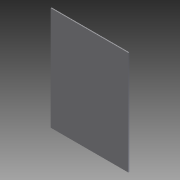
# Autodesk Inventor part: PCB
Saved by Autodesk Inventor 2012 (Build 160160000, 160)
## iProperties
Created: 2017-04-26
Part Number: PCB
Material: Default
Document SubType Name: Modeling
Designer: Brandon
Density: 1 g/cm^3
Author: Brandon
Autodesk Inventor part; units mm, degrees
ref_plane "YZ Plane" through (0, 0, 0) normal (1, 0, 0) x (0, 1, 0)
ref_plane "XZ Plane" through (0, 0, 0) normal (0, 1, 0) x (-1, 0, 0)
ref_plane "XY Plane" through (0, 0, 0) normal (0, 0, 1) x (1, 0, 0)
sketch "Sketch1" plane through (0, 0, 0) normal (0, 0, 1) x (1, 0, 0)
  line L0 (-60, 80) -> (60, 80)
  line L1 (60, 80) -> (60, -80)
  line L2 (60, -80) -> (-60, -80)
  line L3 (-60, -80) -> (-60, 80)
  point P0 (0, 0)
  dimension "d0" = 120
  dimension "d1" = 160
  dimension "d2" = 60
  dimension "d3" = 80
  constraints: 8 end point, 2 parallel, 1 horizontal, 1 perpendicular
  measures "d0" distance of L1.end L2.end
  measures "d1" distance of L0.end L1.end
  measures "d2" distance from line of point (0, 0) L3
  measures "d3" distance from line of L0 point (0, 0)
extrude "Extrusion1" add sketch "Sketch1" along normal blind 1.4732
equation "\"d2\" = 0.5 * d0"
equation "\"d3\" = 0.5 * d1"
body "Solid1"
